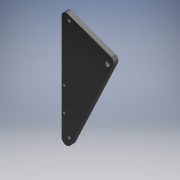
# Autodesk Inventor part: Triangle axle slide connector
Saved by Autodesk Inventor 2019 (Build 230136000, 136)
## iProperties
Part Number: Triangle axle slide connector
Material: Generic
Document SubType Name: Modeling
Designer: Delta
Appearance: Default
Author: Delta
Autodesk Inventor part; units mm, degrees
ref_plane "YZ Plane" through (0, 0, 0) normal (1, 0, 0) x (0, 1, 0)
ref_plane "XZ Plane" through (0, 0, 0) normal (0, 1, 0) x (-1, 0, 0)
ref_plane "XY Plane" through (0, 0, 0) normal (0, 0, 1) x (1, 0, 0)
sketch "Sketch1" plane through (0, 0, 0) normal (0, 0, 1) x (1, 0, 0)
  line L0 (0, 0) -> (0, 177.8)
  line L1 (0, 0) -> (53.8815, 0) construction
  line L2 (0, 177.8) -> (71.6046, 151.7381)
  line L3 (0, 177.8) -> (76.2, 177.8) construction
  line L4 (71.6046, 151.7381) -> (0, 0)
  dimension "d0" = 177.8
  dimension "d19" = 76.2
  dimension "d20" = 20
  constraints: 10 end point, 2 horizontal, 1 equal length, 1 vertical
  measures "d0" distance of L0.start L0.end
  measures "d19" distance of L0.end L2.end
  measures "d20" angle of L2 L3
extrude "Extrusion1" add sketch "Sketch1" along normal blind 6.35
fillet "Fillet1" radius 6.35 2 edges at (0, 177.8, 3.175) (0, 0, 3.175)
sketch "Sketch2" plane through (0, 0, 6.35) normal (0, 0, 1) x (1, 0, 0)
  line L0 (62.618, 177.8) -> (10.16, 177.8) projected
  line L1 (0, 168.7313) -> (0, 28.3357) projected
  circle A0 centre (10.0076, 167.7924) radius 1.905
  circle A1 centre (10.0076, 32.7914) radius 1.905
  circle A2 centre (60.8026, 143.1036) radius 3.175
  point P0 (0, 0)
  dimension "d5" = 10.0076
  dimension "d6" = 10.0076
  dimension "d7" = 10.0076
  dimension "d8" = 135.001
  dimension "d9" = 34.6964
  dimension "d11" = 3.81
  dimension "d12" = 3.81
  dimension "d13" = 6.35
  constraints: 3 centre point, 3 coincident
  measures "d5" distance from line of L0 point (10.008, 167.792)
  measures "d6" distance from line of L1 point (10.008, 167.792)
  measures "d7" distance from line of L1 point (10.008, 32.791)
  measures "d8" distance of point (10.008, 32.791) point (10.008, 167.792)
  measures "d9" distance from line of L0 point (60.803, 143.104)
  measures "d11" diameter of A0
  measures "d12" diameter of A1
  measures "d13" diameter of A2
extrude "Extrusion2" cut sketch "Sketch2" against normal through all
fillet "Fillet4" radius 6.35 1 edges at (71.6046, 151.7381, 3.175)
sketch "Sketch3" plane through (0, 0, 6.35) normal (0, 0, 1) x (1, 0, 0)
  circle A0 centre (3.175, 58.1807) radius 1.651
  circle A1 centre (3.175, 89.9307) radius 1.651
  line L0 (0, 168.7313) -> (0, 28.3357) projected
  point P0 (0, 0)
  dimension "d22" = 3.302
  dimension "d23" = 3.302
  dimension "d24" = 3.175
  dimension "d25" = 3.175
  dimension "d26" = 29.845
  dimension "d27" = 31.75
  constraints: 2 centre point
  measures "d22" diameter of A0
  measures "d23" diameter of A1
  measures "d24" distance from line of L0 A0.centre
  measures "d25" distance from line of L0 A1.centre
  measures "d26" vertical distance of L0.end A0.centre
  measures "d27" distance of A0.centre A1.centre
extrude "Extrusion3" cut sketch "Sketch3" against normal through all
equation "\"d6\" = d5"
equation "\"d7\" = d5"
body "Solid1"
